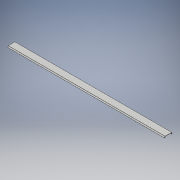
# Autodesk Inventor part: the inside slider part
Saved by Autodesk Inventor 2017 (Build 210142000, 142)
## iProperties
Created: 2019-02-04
Part Number: the inside slider part
Material: Generic
Document SubType Name: Modeling
Designer: S346852600
Density: 1 g/cm^3
Appearance: Default
Author: S346852600
Autodesk Inventor part; units mm, degrees
ref_plane "YZ Plane" through (0, 0, 0) normal (1, 0, 0) x (0, 1, 0)
ref_plane "XZ Plane" through (0, 0, 0) normal (0, 1, 0) x (-1, 0, 0)
ref_plane "XY Plane" through (0, 0, 0) normal (0, 0, 1) x (1, 0, 0)
sketch "Sketch1" plane through (0, 0, 0) normal (1, 0, 0) x (0, 1, 0)
  line L0 (0, -0.4446) -> (0, -37.6554)
  line L1 (-0.4178, 0.1521) -> (-6.7426, 2.4541)
  line L2 (-7.4463, 2.2656) -> (-9.6095, -0.3124)
  line L3 (-0.4178, -38.2521) -> (-6.7426, -40.5541)
  line L4 (-7.4463, -40.3656) -> (-9.6095, -37.7876)
  line L5 (-8.0529, -36.4814) -> (-6.8042, -37.9695)
  line L6 (-6.1006, -38.158) -> (-2.4498, -36.8293)
  line L7 (-2.032, -36.2325) -> (-2.032, -1.8675)
  line L8 (-2.4498, -1.2707) -> (-6.1006, 0.058)
  line L9 (-6.8042, -0.1305) -> (-8.0529, -1.6186)
  line L10 (-9.6095, -0.3124) -> (-8.0529, -1.6186)
  line L11 (-8.0529, -36.4814) -> (-9.6095, -37.7876)
  arc A0 (0, -0.4446) -> (-0.4178, 0.1521) centre (-0.635, -0.4446) ccw
  arc A1 (-2.032, -1.8675) -> (-2.4498, -1.2707) centre (-2.667, -1.8675) ccw
  arc A2 (-6.1006, 0.058) -> (-6.8042, -0.1305) centre (-6.3178, -0.5387) ccw
  arc A3 (-6.7426, 2.4541) -> (-7.4463, 2.2656) centre (-6.9598, 1.8574) ccw
  arc A4 (-0.4178, -38.2521) -> (0, -37.6554) centre (-0.635, -37.6554) ccw
  arc A5 (-2.4498, -36.8293) -> (-2.032, -36.2325) centre (-2.667, -36.2325) ccw
  arc A6 (-6.8042, -37.9695) -> (-6.1006, -38.158) centre (-6.3178, -37.5613) ccw
  arc A7 (-7.4463, -40.3656) -> (-6.7426, -40.5541) centre (-6.9598, -39.9574) ccw
  point P0 (0, 0)
  point P1 (0, -38.1)
  point P2 (-7.1605, 2.6062)
  point P3 (-7.1605, -40.7062)
  point P4 (-6.5184, -38.3101)
  point P5 (-6.5184, 0.2101)
  dimension "d7" = 7.62
  dimension "d8" = 3.81
  dimension "d9" = 110
  dimension "d10" = 110
  dimension "d11" = 7.62
  dimension "d12" = 3.81
  dimension "d13" = 110
  dimension "d14" = 110
  dimension "d15" = 38.1
  dimension "d16" = 2.032
  dimension "d17" = 2.3872
  dimension "d18" = 2.3872
  dimension "d19" = 0.635
  constraints: 24 end point, 16 point on circle, 16 tangent, 12 point on line, 8 centre point, 7 equal radius, 1 vertical, 4 other
  measures "d7" distance of point (0, 0) point (-7.16, 2.606)
  measures "d8" distance of point (-7.16, 2.606) L2.end
  measures "d9" angle of L1 L0
  measures "d10" angle of L1 L2
  measures "d11" distance of point (0, -38.1) point (-7.16, -40.706)
  measures "d12" distance of point (-7.16, -40.706) L4.end
  measures "d13" angle of L3 L0
  measures "d14" angle of L4 L3
  measures "d15" distance of point (0, 0) point (0, -38.1)
  measures "d16" distance between parallel lines of L0 L7
  measures "d17" distance of L5.start point (-6.518, -38.31)
  measures "d18" distance of point (-6.518, 0.21) L9.end
  measures "d19" radius of A0
extrude "Extrusion1" add sketch "Sketch1" along normal blind 878.84
body "Solid1"
